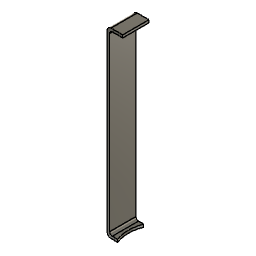
Motor Hook v8 (Autodesk Fusion 360 design; units mm, degrees)
Autodesk Fusion 360 part; units mm, degrees
note: some values were not read from the file. Set by a fixed rule: which sketch regions a step uses.
sketch "Sketch1" plane through (0, 0, 0) normal (0, 1, 0) x (1, 0, 0)
  line L0 (6, -26.7) -> (-2, -26.7)
  line L1 (-1.2679, -27.7) -> (6, -27.7)
  line L2 (6, -27.7) -> (6, -26.7)
  line L3 (-3, -25.7) -> (-3, 40)
  line L4 (-4, 39.268) -> (-4, -26.2)
  line L5 (-2.5, 42) -> (0, 42)
  line L6 (0, 42) -> (0, 41)
  line L7 (0, 41) -> (-2, 41)
  arc A0 (-2, 41) -> (-3, 40) centre (-2, 40) ccw
  arc A1 (-3, -25.7) -> (-2, -26.7) centre (-2, -25.7) ccw
  line L8 (-1.2679, -27.7) -> (-2.5, -27.7)
  line L9 (-4, 39.268) -> (-4, 40.5)
  arc A2 (-2.5, 42) -> (-4, 40.5) centre (-2.5, 40.5) ccw
  arc A3 (-4, -26.2) -> (-2.5, -27.7) centre (-2.5, -26.2) ccw
  dimension "d6" = 67.7
  dimension "d7" = 1
  dimension "d8" = 1
  dimension "d9" = 1
  dimension "d12" = 10
  dimension "d13" = 1.5
  dimension "d14" = 1.5
  constraint horizontal L0
  constraint horizontal L1
  constraint vertical L2
  constraint vertical L3
  constraint vertical L4
  constraint horizontal L5
  constraint vertical L6
  constraint horizontal L7
  constraint tangent L3 A0
  constraint tangent L7 A0
  constraint tangent L0 A1
  constraint tangent L3 A1
  constraint perpendicular L4 L8
  constraint perpendicular L5 L9
  constraint tangent L5 A2
  constraint tangent L9 A2
  constraint tangent L8 A3
  constraint tangent L4 A3
  measures "d6" distance of L0 L7
  measures "d7" distance of L0 L1
  measures "d8" distance of L3 L4
  measures "d9" distance of L5 L7
  measures "d12" distance of L2 L4
  measures "d13" radius of A2
  measures "d14" radius of A3
extrude "Extrude1" add sketch "Sketch1" along normal blind 10
sketch "Sketch2" plane through (0, 0, -41) normal (0, 0, 1) x (-1, 0, 0)
  line L0 (2, 0) -> (0, 0)
  line L1 (0, 0) -> (0, -10)
  line L2 (0, -10) -> (2, -10)
  line L3 (2, -10) -> (2, 0)
  line L4 (0, 0) -> (0, -10)
  line L5 (-13.3846, -5) -> (0, -10) construction
  line L6 (-13.3846, -5) -> (0, 0) construction
  arc A0 (0, -10) -> (0, 0) centre (-13.3846, -5) ccw
  arc A1 (0, -10) -> (0, 0) centre (-13.3846, -5) ccw
  dimension "d19" = 14.288
  dimension "d20" = 14.288
  constraint coincident L1.end L2.start
  constraint coincident L0.end L1.start
  constraint coincident L5.start L6.start
  measures "d19" distance of L5.start L1.end
  measures "d20" distance of L0.end L5.start
extrude "Extrude2" cut sketch "Sketch2" against normal blind 10 contours L1 L4 A0 A1
extrude "Extrude3" cut 1 faces at (6, 3.3333, 27.3667) along direction (-1, 0, 0) blind 4
equation "d6 = 80 mm - 12.3 mm"
